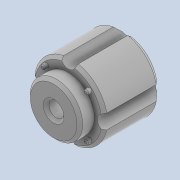
# Autodesk Inventor part: centrifugetool_5mm_base_v2
Saved by Autodesk Inventor 2021.2 (Build 252289000, 289)
## iProperties
Created: 2021-10-27
Part Number: centrifugetool_5mm_base_v2
Material: Generic
Document SubType Name: Modeling
Designer: to172
Density: 1 g/cm^3
Appearance: Smooth - Medium Gray
Author: to172
Autodesk Inventor part; units mm, degrees
ref_plane "YZ Plane" through (0, 0, 0) normal (1, 0, 0) x (0, 1, 0)
ref_plane "XZ Plane" through (0, 0, 0) normal (0, 1, 0) x (-1, 0, 0)
ref_plane "XY Plane" through (0, 0, 0) normal (0, 0, 1) x (1, 0, 0)
sketch "Sketch1" plane through (0, 0, 0) normal (0, 0, 1) x (1, 0, 0)
  circle A0 centre (0, 0) radius 12.5
  dimension "d0" = 25
  constraints: 1 centre point, 1 coincident
  measures "d0" diameter of A0
extrude "Extrusion1" add sketch "Sketch1" along normal blind 25
chamfer "Chamfer2" distance 2 angle 45 1 edges at (-12.5, 0, 0)
sketch "Sketch2" plane through (0, 0, 0) normal (1, 0, 0) x (0, 1, 0)
  line L0 (0, 0) -> (1, 0)
  line L1 (1, 0) -> (1, 4)
  line L2 (1, 4) -> (0, 4)
  line L3 (0, 4) -> (0, 0)
  line L4 (12.5, 25) -> (-12.5, 25) projected
  line L5 (0, 4) -> (2.575, 4)
  line L6 (2.575, 4) -> (2.575, 25)
  line L7 (2.575, 25) -> (0, 25)
  line L8 (0, 25) -> (0, 4)
  line L9 (2.575, 4) -> (1, 2.685)
  line L10 (1, 2.685) -> (0, 1.85) construction
  dimension "d9" = 1
  dimension "d10" = 2.575
  dimension "d11" = 4
  dimension "d42" = 2.15
  constraints: 20 end point, 4 parallel, 4 point on line, 2 horizontal, 2 perpendicular
  measures "d9" distance between parallel lines of L3 L1
  measures "d10" distance between parallel lines of L8 L6
  measures "d11" distance between parallel lines of L0 L5
  measures "d42" vertical distance of L5.end L10.end
revolve "Revolution1" cut sketch "Sketch2" angle 360 about axis through (0, 0, 25) along (0, 0, -1)
chamfer "Chamfer3" distance 1 angle 45 2 edges at (0, -1, 0) (0, -2.575, 25)
sketch "Sketch3" plane through (0, 0, 25) normal (0, 0, 1) x (1, 0, 0)
  circle A0 centre (0, 0) radius 9
  line L0 (0, 0) -> (26.029, 0) construction
  circle A1 centre (0, 0) radius 12.5 construction
  circle A2 centre (12.5, 0) radius 2.5
  circle A3 centre (0, 12.5) radius 2.5
  circle A4 centre (-12.5, 0) radius 2.5
  circle A5 centre (0, -12.5) radius 2.5
  circle A6 centre (0, 0) radius 12.5
  point P0 (-2.4875, 12.25)
  point P1 (-12.25, 2.4875)
  point P2 (-12.25, -2.4875)
  point P3 (-2.4875, -12.25)
  point P4 (2.4875, -12.25)
  point P5 (12.25, -2.4875)
  point P6 (12.25, 2.4875)
  point P7 (2.4875, 12.25)
  dimension "d16" = 5
  dimension "d19" = 360
  dimension "d21" = 25
  dimension "d22" = 18
  constraints: 6 centre point, 2 coincident, 2 end point, 1 horizontal, 1 horizontal alignment, 1 point on line, 10 other
  measures "d16" diameter of A2
  measures "d21" diameter of A6
  measures "d22" diameter of A0
extrude "Extrusion2" cut sketch "Sketch3" against normal through all contours A2 A6 | A6 A2 | A6 A3 | A3 A6 | A6 A5 | A5 A6 | A6 A4 | A4 A6
extrude "Extrusion3" cut sketch "Sketch3" against normal blind 5 contours A2 A6 A5 A4 A3
chamfer "Chamfer4" distance 1 angle 45 5 edges at (-9, 0, 25) (-8.8388, -8.8388, 20) (8.8388, -8.8388, 20) (8.8388, 8.8388, 20) (-8.8388, 8.8388, 20)
sketch "Sketch4" plane through (0, 0, 20) normal (0, 0, 1) x (1, 0, 0)
  line L0 (0, 0) -> (-18.6595, 0) construction
  line L1 (0, 0) -> (0, 25.4609) construction
  circle A0 centre (0, 0) radius 2.575 construction
  line L2 (0, 0) -> (-16.5294, 16.5294) construction
  circle A1 centre (-7.4246, 7.4246) radius 0.75
  circle A2 centre (0, 0) radius 3.575 construction
  circle A3 centre (0, 0) radius 10.5 construction
  circle A4 centre (-7.4246, -7.4246) radius 0.75
  circle A5 centre (7.4246, -7.4246) radius 0.75
  circle A6 centre (7.4246, 7.4246) radius 0.75
  point P0 (0, 0)
  dimension "d31" = 21
  dimension "d30" = 45
  dimension "d32" = 1.5
  dimension "d35" = 360
  constraints: 6 end point, 4 centre point, 1 coincident, 1 horizontal, 1 point on line, 1 vertical, 12 other
  measures "d30" angle of L2 L0
  measures "d32" diameter of A1
extrude "Extrusion4" add sketch "Sketch4" along normal blind 1.5
chamfer "Chamfer5" distance 0.35 angle 45 4 edges at (6.6746, 7.4246, 21.5) (-8.1746, 7.4246, 21.5) (-8.1746, -7.4246, 21.5) (6.6746, -7.4246, 21.5)
body "Solid1"
